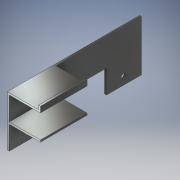
# Autodesk Inventor part: side
Saved by Autodesk Inventor 2016 (Build 200138000, 138)
## iProperties
Created: 2015-10-31
Part Number: side
Material: Generic
Document SubType Name: Modeling
Designer: rossmosier
Density: 1 g/cm^3
Appearance: Chrome - Polished
Author: rossmosier
Autodesk Inventor part; units mm, degrees
ref_plane "YZ Plane" through (0, 0, 0) normal (1, 0, 0) x (0, 1, 0)
ref_plane "XZ Plane" through (0, 0, 0) normal (0, 1, 0) x (-1, 0, 0)
ref_plane "XY Plane" through (0, 0, 0) normal (0, 0, 1) x (1, 0, 0)
sketch "Sketch1" plane through (0, 0, 0) normal (0, 1, 0) x (-1, 0, 0)
  line L0 (0, 0) -> (-88.9, 0)
  line L1 (-88.9, -114.3) -> (-88.9, -317.5)
  line L2 (-88.9, -431.8) -> (0, -431.8)
  line L3 (0, -431.8) -> (0, 0)
  line L4 (-88.9, 0) -> (-165.1, 0)
  line L5 (-165.1, 0) -> (-165.1, -114.3)
  line L6 (-165.1, -114.3) -> (-88.9, -114.3)
  line L7 (-88.9, -114.3) -> (-88.9, 0)
  line L8 (-88.9, -431.8) -> (-165.1, -431.8)
  line L9 (-165.1, -431.8) -> (-165.1, -317.5)
  line L10 (-165.1, -317.5) -> (-88.9, -317.5)
  line L11 (-88.9, -317.5) -> (-88.9, -431.8)
  line L12 (-88.9, -374.65) -> (-139.7, -374.65) construction
  line L13 (-88.9, -58.8342) -> (-139.7, -58.8342) construction
  circle A0 centre (-139.7, -58.8342) radius 7.9375
  circle A1 centre (-139.7, -374.65) radius 7.9375
  dimension "d0" = 88.9
  dimension "d1" = 431.8
  dimension "d2" = 76.2
  dimension "d3" = 114.3
  dimension "d4" = 76.2
  dimension "d5" = 114.3
  dimension "d6" = 50.8
  dimension "d7" = 15.875
  dimension "d8" = 15.875
  constraints: 28 end point, 6 parallel, 5 horizontal, 3 perpendicular, 2 centre point, 2 coincident, 1 midpoint, 1 point on line
  measures "d0" distance of L2.end L2.start
  measures "d1" distance of L2.start L0.end
  measures "d2" distance of L1.start L5.end
  measures "d3" distance of L5.end L4.end
  measures "d4" distance of L1.end L9.end
  measures "d5" distance of L8.end L9.end
  measures "d6" distance of L12.start L12.end
  measures "d7" diameter of A0
  measures "d8" diameter of A1
extrude "Extrusion1" add sketch "Sketch1" along normal blind 6.35
sketch "Sketch6" plane through (0, 0, 0) normal (0, -1, 0) x (1, 0, 0)
  circle A0 centre (139.7, -58.8342) radius 7.9375 projected
  circle A1 centre (139.7, -374.65) radius 7.9375 projected
  line L0 (165.1, -431.8) -> (0, -431.8) projected
  line L1 (165.1, -317.5) -> (165.1, -431.8) projected
  line L2 (88.9, -317.5) -> (165.1, -317.5) projected
  line L3 (88.9, -114.3) -> (88.9, -317.5) projected
  line L4 (165.1, -114.3) -> (88.9, -114.3) projected
  line L5 (165.1, 0) -> (165.1, -114.3) projected
  line L6 (0, 0) -> (165.1, 0) projected
  line L7 (0, -431.8) -> (0, 0) projected
  line L8 (0, -431.8) -> (6.35, -431.8)
  line L9 (6.35, -431.8) -> (6.35, -279.4)
  line L10 (6.35, -279.4) -> (0, -279.4)
  line L11 (0, -279.4) -> (0, -431.8)
  line L12 (88.9, -431.8) -> (82.55, -431.8)
  line L13 (82.55, -431.8) -> (82.55, -279.4)
  line L14 (82.55, -279.4) -> (88.9, -279.4)
  line L15 (88.9, -279.4) -> (88.9, -431.8)
  dimension "d20" = 6.35
  dimension "d21" = 152.4
  constraints: 16 end point, 4 parallel, 2 horizontal, 2 perpendicular, 1 point on line
  measures "d20" distance of L10.end L9.end
  measures "d21" distance of L9.end L8.end
extrude "Extrusion5" add sketch "Sketch6" along normal blind 101.6 contours L0 L13 L14 L3 L15 | L0 L7 L10 L9
sketch "Sketch7" plane through (0, 6.35, -431.8) normal (-1, 0, 0) x (0, 0, 1)
  line L0 (152.4, -6.35) -> (431.8, -6.35) projected
  line L1 (431.8, -6.35) -> (431.8, 0) projected
  line L2 (0, 0) -> (431.8, 0) projected
  line L3 (0, -107.95) -> (0, 0) projected
  line L4 (152.4, -107.95) -> (0, -107.95) projected
  line L5 (152.4, -6.35) -> (152.4, -107.95) projected
  line L6 (152.4, -6.35) -> (152.4, -107.95) projected
  line L7 (0, -107.95) -> (152.4, -107.95)
  line L8 (152.4, -107.95) -> (152.4, -101.6)
  line L9 (152.4, -101.6) -> (0, -101.6)
  line L10 (0, -101.6) -> (0, -107.95)
  dimension "d24" = 6.35
  constraints: 8 end point, 2 parallel, 1 horizontal, 1 perpendicular, 1 point on line
  measures "d24" distance of L8.end L7.end
extrude "Extrusion6" add sketch "Sketch7" along normal blind 12.7 contours L5 L4 L3 L9
body "Solid1"
